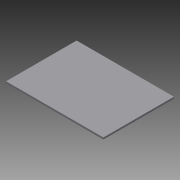
# Autodesk Inventor part: bottom_board
Saved by Autodesk Inventor 2014 SP1 (Build 180222100, 222)
## iProperties
Created: 2014-02-20
Part Number: bottom_board
Material: Wood (Birch)
Document SubType Name: Modeling
Designer: Chris
Density: 0.55 g/cm^3
Appearance: Birch - Natural Polished
Mass: 1119.78 g
Surface Area: 4453.42 cm^2
Volume: 2035.96 cm^3
Author: Chris
Autodesk Inventor part; units mm, degrees
ref_plane "YZ Plane" through (0, 0, 0) normal (1, 0, 0) x (0, 1, 0)
ref_plane "XZ Plane" through (0, 0, 0) normal (0, 1, 0) x (-1, 0, 0)
ref_plane "XY Plane" through (0, 0, 0) normal (0, 0, 1) x (1, 0, 0)
sketch "Sketch1" plane through (0, 0, 0) normal (0, 0, 1) x (1, 0, 0)
  line L0 (-166.6875, 88.7016) -> (376.2375, 88.7016)
  line L1 (376.2375, 88.7016) -> (376.2375, 79.1766)
  line L2 (376.2375, 79.1766) -> (-166.6875, 79.1766)
  line L3 (-166.6875, 79.1766) -> (-166.6875, 88.7016)
  point P0 (0, 0)
  dimension "d0" = 542.925
  dimension "d1" = 9.525
  constraints: 8 end point, 2 parallel, 1 horizontal, 1 perpendicular
  measures "d0" distance of L0.start L0.end
  measures "d1" distance of L2.end L0.start
extrude "Extrusion1" add sketch "Sketch1" against normal blind 393.7
body "Solid1"
